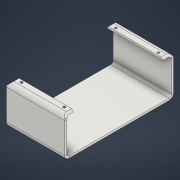
# Autodesk Inventor part: puszka
Saved by Autodesk Inventor 2021 (Build 250183000, 183)
## iProperties
Created: 2021-03-29
Part Number: puszka
Material: Stal
Document SubType Name: Konstrukcja blachowa
Designer: Karol
Density: 7.85 g/cm^3
Sheet Metal Rule: Domyślny_mm
Appearance: Stal
Flat Pattern Width: 6 cm
Flat Pattern Length: 19.7237 cm
Flat Pattern Area: 118.342 cm^2
Sheet Metal Width: 60,000 mm
Sheet Metal Length: 197,237 mm
Sheet Metal Area: 11834,230 mm^2
Author: Karol
Autodesk Inventor part; units mm, degrees
ref_plane "YZ Plane" through (0, 0, 0) normal (1, 0, 0) x (0, 1, 0)
ref_plane "XZ Plane" through (0, 0, 0) normal (0, 1, 0) x (-1, 0, 0)
ref_plane "XY Plane" through (0, 0, 0) normal (0, 0, 1) x (1, 0, 0)
sketch "Szkic1" plane through (0, 0, 0) normal (0, 1, 0) x (-1, 0, 0)
  line L0 (-30, 56) -> (30, 56)
  line L1 (30, 56) -> (30, -56)
  line L2 (30, -56) -> (-30, -56)
  line L3 (-30, -56) -> (-30, 56)
  line L4 (-30, 56) -> (30, -56) construction
  line L5 (30, 56) -> (-30, -56) construction
  point P0 (0, 0)
  dimension "d0" = 60
  dimension "d1" = 112
  measures "d0" distance of L1.end L2.end
  measures "d1" distance of L0.end L1.end
extrude "Płyta1" add sketch "Szkic1" along normal blind 2
sketch "Szkic2" plane through (30, 0, 54) normal (0, 0, 1) x (1, 0, 0)
  line L0 (-60, 0) -> (0, 0)
  line L1 (0, 0) -> (0, 40)
  line L2 (0, 40) -> (-60, 40)
  line L3 (-60, 40) -> (-60, 0)
  constraints: 6 end point, 1 horizontal, 1 perpendicular, 1 vertical
edge flange "Kołnierz1" height 40 angle 90 thickness 2 bend radius 2.5 thickness toward (0, 0, 1) relief tear relief width 2 relief depth 1 corner gap 2 corner form 0 edges at (0, 2, 56) (0, 2, -56) wall of the first edge with corners at (-30, 0, 54) (30, 0, 54) (30, 40, 54) (-30, 40, 54)
bend "Zagięcie1"
corner "Narożnik1"
sketch "Szkic3" plane through (30, 38, 56) normal (0, 1, 0) x (-1, 0, 0)
  line L0 (60, 0) -> (0, 0)
  line L1 (0, 0) -> (0, -10)
  line L2 (0, -10) -> (60, -10)
  line L3 (60, -10) -> (60, 0)
  constraints: 6 end point, 1 horizontal, 1 perpendicular, 1 vertical
edge flange "Kołnierz2" height 10 angle 90 thickness 2 bend radius 2.5 thickness toward (0, 1, 0) relief tear relief width 2 relief depth 1 corner gap 2 corner form 0 edges at (0, 40, 54) (0, 40, -54) wall of the first edge with corners at (-30, 38, 56) (30, 38, 56) (30, 38, 46) (-30, 38, 46)
bend "Zagięcie2"
corner "Narożnik2"
sketch "Szkic4" plane through (-30, 40, 46) normal (0, 1, 0) x (1, 0, 0)
  line L0 (60, 92) -> (0, 92) projected
  line L1 (0, 0) -> (60, 0) projected
  line L2 (0, 92) -> (0, 97.5) projected
  line L3 (60, 97.5) -> (60, 92) projected
  point P0 (30, 46)
  point P1 (8, -2.5)
  point P2 (52, -2.5)
  point P3 (8, 94.5)
  point P4 (52, 94.5)
  dimension "d24" = 2.5
  dimension "d25" = 2.5
  dimension "d26" = 2.5
  dimension "d27" = 2.5
  dimension "d28" = 8
  dimension "d29" = 8
  constraints: 2 vertical alignment
  measures "d24" distance from line of L0 point (8, 94.5)
  measures "d25" distance from line of L0 point (52, 94.5)
  measures "d26" distance from line of L1 point (8, -2.5)
  measures "d27" distance from line of L1 point (52, -2.5)
  measures "d28" distance from line of L2 point (8, 94.5)
  measures "d29" distance from line of L3 point (52, 94.5)
hole "Otwór1" at (-22, 40, 48.5) at (22, 40, 48.5) at (-22, 40, -48.5) at (22, 40, -48.5) direction (0, -1, 0) diameter 2.459 depth 8.8 tip angle 118 thread size "M3x0.5" class "6H" standard "ANSI Metric M Profile"
sketch "Szkic5" plane through (30, 4.5, -56) normal (0, 0, -1) x (-1, 0, 0)
  line L0 (0, 33.5) -> (0, 31) projected
  line L1 (0, 32.5) -> (3, 35.5)
  line L2 (0, 35.5) -> (60, 35.5) projected
  line L3 (0, 35.5) -> (0, 31) projected
  point P0 (30, -4.5)
  dimension "d37" = 45
  dimension "d38" = 3
  constraints: 2 end point, 2 point on line
  measures "d37" angle of L3 L1
  measures "d38" distance from line of L2 L1.start
extrude "Wyciągnięcie proste1" cut sketch "Szkic5" against normal through all
mirror "Odbij1" about plane through (0, 0, 0) normal (1, 0, 0) of "Wyciągnięcie proste1"
equation "\"d2\" = Grubość"
equation "\"d3\" = SzerokośćGięciaPodcięcia"
equation "\"d4\" = GłębokośćGięciaPodcięcia"
equation "\"d5\" = MinimalnaPozostałość"
equation "\"d6\" = PromieńPrzejścia"
equation "\"d10\" = RozmiarPodcięciaNarożnika"
equation "\"d11\" = Wielk_odstępu"
equation "\"d12\" = Rozmiar_promienia_Jacobiego"
equation "\"d14\" = SzerokośćGięciaPodcięcia"
equation "\"d15\" = GłębokośćGięciaPodcięcia"
equation "\"d16\" = MinimalnaPozostałość"
equation "\"d17\" = PromieńPrzejścia"
equation "\"d21\" = RozmiarPodcięciaNarożnika"
equation "\"d22\" = Wielk_odstępu"
equation "\"d23\" = Rozmiar_promienia_Jacobiego"
equation "\"PromieńGięcia\" = Grubość"
equation "\"SzerokośćGięciaPodcięcia\" = Grubość"
equation "\"GłębokośćGięciaPodcięcia\" = 0.5 * Grubość"
equation "\"RozmiarPodcięciaNarożnika\" = 4 * Grubość"
equation "\"MinimalnaPozostałość\" = 2 * Grubość"
equation "\"PromieńPrzejścia\" = PromieńGięcia"
equation "\"Rozmiar_promienia_Jacobiego\" = PromieńGięcia"
equation "\"Wielk_odstępu\" = Grubość"
equation "\"Grubość\" = 2"
